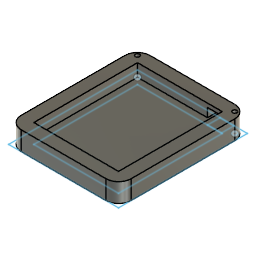
case (Autodesk Fusion 360 design; units mm, degrees)
part number: 2026-03-26-22-18-51-213
Autodesk Fusion 360 part; units mm, degrees
note: some values were not read from the file. Chosen so that the rebuilt part matches the saved one: that a step has no effect.
sketch "Szkic1" plane through (0, 0, 0) normal (0, 0, 1) x (1, 0, 0)
  line L0 (-35, 30, 10) -> (32, 30, 10)
  line L1 (32, 30, 10) -> (32, -52, 10)
  line L2 (32, -52, 10) -> (-35, -52, 10)
  line L3 (-35, -52, 10) -> (-35, 30, 10)
  line L4 (-45, 40, 10) -> (42, 40, 10)
  line L5 (42, 40, 10) -> (42, -62, 10)
  line L6 (42, -62, 10) -> (-45, -62, 10)
  line L7 (-45, -62, 10) -> (-45, 40, 10)
  circle A0 through (-38.3, 35, 10) (-40.85, 36.4722, 10) (-40.85, 33.5278, 10)
  circle A1 through (38.7, 35, 10) (36.15, 36.4722, 10) (36.15, 33.5278, 10)
  line L8 (20.4, 40, 10) -> (31.4, 40, 10)
  line L9 (31.4, 40, 10) -> (31.4, 30, 10)
  line L10 (31.4, 30, 10) -> (20.4, 30, 10)
  line L11 (20.4, 30, 10) -> (20.4, 40, 10)
  dimension "d1" = 67
  dimension "d2" = 82
  dimension "d3" = 87
  dimension "d4" = 102
  dimension "d5" = 10
  dimension "d6" = 10
  dimension "d15" = 3.4
  dimension "d16" = 5
  dimension "d17" = 5
  dimension "d18" = 3.4
  dimension "d19" = 5
  dimension "d20" = 5
  dimension "d30" = 0.6
  dimension "d31" = 11
sketch "Szkic1 (curves 10 mm off its plane)" plane through (0, 0, 10) normal (0, 0, 1) x (1, 0, 0)
  line L0 (-35, 30) -> (32, 30)
  line L1 (32, 30) -> (32, -52)
  line L2 (32, -52) -> (-35, -52)
  line L3 (-35, -52) -> (-35, 30)
  line L4 (-45, 40) -> (42, 40)
  line L5 (42, 40) -> (42, -62)
  line L6 (42, -62) -> (-45, -62)
  line L7 (-45, -62) -> (-45, 40)
  circle A0 centre (-40, 35) radius 1.7
  circle A1 centre (37, 35) radius 1.7
  line L8 (20.4, 40) -> (31.4, 40)
  line L9 (31.4, 40) -> (31.4, 30)
  line L10 (31.4, 30) -> (20.4, 30)
  line L11 (20.4, 30) -> (20.4, 40)
extrude "Wyciągnięcie proste1" add sketch "Szkic1 (curves 10 mm off its plane)" along normal blind 5 contours L0 L1 L2 L3 L10
extrude "Wyciągnięcie proste2" add sketch "Szkic1 (curves 10 mm off its plane)" along normal blind 15 contours L0 L1 L2 L3 L4 L5 L6 L7 L9 L11 | L0 L4 L8 L9 L10 L11 | A0 | A1
fillet "Zaokrąglenie1" radius 10 4 edges at (-45, -62, 17.5) (42, -62, 17.5) (42, 40, 17.5) (-45, 40, 17.5)
extrude "Wyciągnięcie proste3" [no effect]
extrude "Wyciągnięcie proste4" cut sketch "Szkic1 (curves 10 mm off its plane)" along normal blind 17 and the other way blind -10 contours A0
extrude "Wyciągnięcie proste5" cut sketch "Szkic1 (curves 10 mm off its plane)" along normal blind 18 and the other way blind -10 contours A1
extrude "Wyciągnięcie proste6" cut sketch "Szkic1 (curves 10 mm off its plane)" along normal blind 12 and the other way blind -5 contours L0 L4 L8 L9 L10 L11
